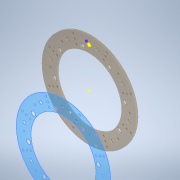
# Autodesk Inventor part: IntakeCCenterWheelInterposer
Saved by Autodesk Inventor 2020 (Build 240168000, 168)
## iProperties
Created: 2020-01-19
Part Number: IntakeCCenterWheelInterposer
Material: Generic
Document SubType Name: Modeling
Designer: srini
Density: 1 g/cm^3
Appearance: Polycarbonate - Smoked
Author: srini
Autodesk Inventor part; units mm, degrees
ref_plane "YZ Plane" through (0, 0, 0) normal (1, 0, 0) x (0, 1, 0)
ref_plane "XZ Plane" through (0, 0, 0) normal (0, 1, 0) x (-1, 0, 0)
ref_plane "XY Plane" through (0, 0, 0) normal (0, 0, 1) x (1, 0, 0)
sketch "Sketch1" plane through (0, 0, 0) normal (0, 0, 1) x (1, 0, 0)
  circle A0 centre (0, 0) radius 98.425
  circle A1 centre (0, 0) radius 142.875
  dimension "d0" = 196.85
  dimension "d1" = 44.45
  constraints: 2 centre point, 2 coincident
  measures "d0" diameter of A0
  measures "d1" radial gap between concentric circles of A0 A1
extrude "Extrusion1" add sketch "Sketch1" along normal blind 6.35
sketch "Sketch2" plane through (0, 0, 6.35) normal (0, 0, 1) x (1, 0, 0)
  circle A0 centre (0, 120.269) radius 2.5797
  line L0 (0, 120.269) -> (0, 0) construction
  line L1 (0, 0) -> (23.4633, 117.9581) construction
  line L2 (0, 0) -> (51.0308, 123.1993) construction
  line L3 (0, 0) -> (63.5017, 95.037) construction
  circle A1 centre (23.4633, 117.9581) radius 4.445
  circle A2 centre (-85.043, 85.043) radius 2.5797
  circle A3 centre (-66.8179, 100) radius 4.445
  circle A4 centre (-120.269, 0) radius 2.5797
  circle A5 centre (-117.9581, 23.4633) radius 4.445
  circle A6 centre (-85.043, -85.043) radius 2.5797
  circle A7 centre (-100, -66.8179) radius 4.445
  circle A8 centre (0, -120.269) radius 2.5797
  circle A9 centre (-23.4633, -117.9581) radius 4.445
  circle A10 centre (85.043, -85.043) radius 2.5797
  circle A11 centre (66.8179, -100) radius 4.445
  circle A12 centre (120.269, 0) radius 2.5797
  circle A13 centre (117.9581, -23.4633) radius 4.445
  circle A14 centre (85.043, 85.043) radius 2.5797
  circle A15 centre (100, 66.8179) radius 4.445
  circle A16 centre (51.0308, 123.1993) radius 2.5797
  circle A17 centre (46.1708, 111.4661) radius 2.5797
  circle A18 centre (41.3107, 99.7328) radius 2.5797
  circle A19 centre (59.9738, 89.7571) radius 6.35
  line L4 (59.9738, 89.7571) -> (0, 0)
  circle A20 centre (-21.06, 105.8758) radius 6.35
  circle A21 centre (-89.7571, 59.9738) radius 6.35
  circle A22 centre (-105.8758, -21.06) radius 6.35
  circle A23 centre (-59.9738, -89.7571) radius 6.35
  circle A24 centre (21.06, -105.8758) radius 6.35
  circle A25 centre (89.7571, -59.9738) radius 6.35
  circle A26 centre (105.8758, 21.06) radius 6.35
  circle A27 centre (-41.3107, 99.7328) radius 2.5797
  circle A28 centre (-46.1708, 111.4661) radius 2.5797
  circle A29 centre (-51.0308, 123.1993) radius 2.5797
  circle A30 centre (-99.7328, 41.3107) radius 2.5797
  circle A31 centre (-111.4661, 46.1708) radius 2.5797
  circle A32 centre (-123.1993, 51.0308) radius 2.5797
  circle A33 centre (-99.7328, -41.3107) radius 2.5797
  circle A34 centre (-111.4661, -46.1708) radius 2.5797
  circle A35 centre (-123.1993, -51.0308) radius 2.5797
  circle A36 centre (-41.3107, -99.7328) radius 2.5797
  circle A37 centre (-46.1708, -111.4661) radius 2.5797
  circle A38 centre (-51.0308, -123.1993) radius 2.5797
  circle A39 centre (41.3107, -99.7328) radius 2.5797
  circle A40 centre (46.1708, -111.4661) radius 2.5797
  circle A41 centre (51.0308, -123.1993) radius 2.5797
  circle A42 centre (99.7328, -41.3107) radius 2.5797
  circle A43 centre (111.4661, -46.1708) radius 2.5797
  circle A44 centre (123.1993, -51.0308) radius 2.5797
  circle A45 centre (99.7328, 41.3107) radius 2.5797
  circle A46 centre (111.4661, 46.1708) radius 2.5797
  circle A47 centre (123.1993, 51.0308) radius 2.5797
  circle A48 centre (0, 133.35) radius 2.5797
  circle A49 centre (-94.2927, 94.2927) radius 2.5797
  circle A50 centre (-133.35, 0) radius 2.5797
  circle A51 centre (-94.2927, -94.2927) radius 2.5797
  circle A52 centre (0, -133.35) radius 2.5797
  circle A53 centre (94.2927, -94.2927) radius 2.5797
  circle A54 centre (133.35, 0) radius 2.5797
  circle A55 centre (94.2927, 94.2927) radius 2.5797
  dimension "d4" = 5.1594
  dimension "d5" = 120.269
  dimension "d6" = 11.25
  dimension "d7" = 22.5
  dimension "d8" = 33.75
  dimension "d9" = 8.89
  dimension "d12" = 360
  dimension "d14" = 133.35
  dimension "d17" = 12.7
  dimension "d22" = 114.3
  dimension "d36" = 12.7
  dimension "d37" = 107.95
  dimension "d38" = 33.75
  dimension "d41" = 360
  dimension "d45" = 360
  dimension "d47" = 133.35
  dimension "d50" = 360
  constraints: 56 centre point, 33 coincident, 10 end point, 2 equal radius, 1 equal length, 1 point on line, 1 vertical, 155 other
  measures "d4" diameter of A0
  measures "d5" distance of L0.start L0.end
  measures "d6" angle of L1 L0
  measures "d7" angle of L2 L0
  measures "d8" angle of L3 L0
  measures "d9" diameter of A1
  measures "d14" distance of L0.end L2.end
  measures "d17" distance of L2.end point (46.171, 111.466)
  measures "d22" distance of L0.end L3.end
  measures "d36" diameter of A19
  measures "d37" distance of L4.start L0.end
  measures "d38" angle of L4 L0
  measures "d47" distance of point (0, 0) A48.centre
extrude "Extrusion2" cut sketch "Sketch2" against normal blind 6.35 contours A0 | A1 | A2 | A3 | A4 | A5 | A6 | A7 | A8 | A9 | A10 | A11 | A12 | A13 | A14 | A15 | A16 | A17 | A18 | A19 | A20 | A21 | A22 | A23 | A24 | A25 | A26 | A27 | A28 | A29 | A30 | A31 | A32 | A33 | A34 | A35 | A36 | A37 | A38 | A39 | A40 | A41 | A42 | A43 | A44 | A45 | A46 | A47
equation "\"d38\" = d8"
equation "\"d47\" = d14"
body "Solid1"
